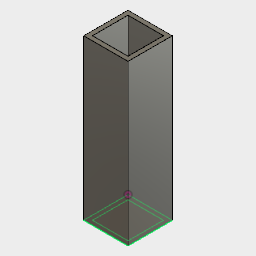
Cuvette (Autodesk Fusion 360 design; units mm, degrees)
Autodesk Fusion 360 part; units mm, degrees
sketch "Sketch1" plane through (0, 0, 0) normal (0, 1, 0) x (1, 0, 0)
  line L0 (0, 0) -> (12.5, 0)
  line L1 (12.5, 0) -> (12.5, -12.5)
  line L2 (12.5, -12.5) -> (0, -12.5)
  line L3 (0, -12.5) -> (0, 0)
  line L4 (11.25, -11.25) -> (1.25, -11.25)
  line L5 (1.25, -11.25) -> (1.25, -1.25)
  line L6 (1.25, -1.25) -> (11.25, -1.25)
  line L7 (11.25, -1.25) -> (11.25, -11.25)
  dimension "d1" = 12.5
  dimension "d2" = 90
  dimension "d3" = 12.5
  dimension "d4" = 1.25
  measures "d1" distance of L0.start L0.end
  measures "d2" angle of L0 L3
  measures "d3" distance of L0.start L2.end
extrude "Extrude1" add sketch "Sketch1" along normal blind 1 contours L4 L5 L6 L7
extrude "Extrude2" add sketch "Sketch1" along normal blind 45
